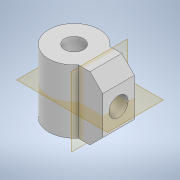
# Autodesk Inventor part: joint
Saved by Autodesk Inventor 2021 (Build 250183000, 183)
## iProperties
Created: 2020-12-08
Part Number: joint
Material: Generic
Document SubType Name: Modeling
Designer: awitc
Density: 1 g/cm^3
Appearance: Default
Author: awitc
Autodesk Inventor part; units mm, degrees
ref_plane "XY Plane" through (0, 0, 0) normal (0, 0, 1) x (1, 0, 0)
sketch "Sketch1" plane through (0, 0, 0) normal (0, 1, 0) x (-1, 0, 0)
  circle A0 centre (0, 0) radius 4
  circle A1 centre (0, 0) radius 1.5
  dimension "d0" = 8
  dimension "d1" = 3
  constraints: 2 centre point, 2 coincident
  measures "d0" diameter of A0
  measures "d1" diameter of A1
extrude "Extrusion1" add sketch "Sketch1" along normal blind 10
ref_plane "Work Plane1" through (4, 0, 0) normal (1, 0, 0) x (0, 1, 0)
sketch "Sketch2" plane through (4, 0, 0) normal (1, 0, 0) x (0, 1, 0)
  line L0 (0, -4) -> (10, -4) projected
  line L1 (10, -4) -> (10, 4) projected
  line L2 (0, -4) -> (10, -4)
  line L3 (10, -4) -> (10, 4)
  line L4 (10, 4) -> (0, 4)
  line L5 (0, 4) -> (0, -4)
  line L6 (0, 0) -> (0, 2.5)
  line L7 (0, -4) -> (0, 4) projected
  line L8 (0, 2.5) -> (0, -2.5)
  line L9 (0, -2.5) -> (10, -2.5)
  line L10 (0, 2.5) -> (10, 2.5)
  dimension "d5" = 2.5
  dimension "d6" = 5
  constraints: 16 end point, 5 point on line, 3 perpendicular, 2 parallel, 1 horizontal
  measures "d5" distance of L6.start L6.end
  measures "d6" distance of L6.end L8.end
extrude "Extrusion2" add sketch "Sketch2" along normal blind 3 and the other way blind 2.5 contours L5 L10 L1 L9
sketch "Sketch3" plane through (7, 0, 0) normal (1, 0, 0) x (0, 0, -1)
  line L0 (0, 0) -> (0, 10)
  line L1 (4, 10) -> (-4, 10) projected
  circle A0 centre (0, 5) radius 1.5
  point P0 (2.5, 10)
  point P1 (-2.5, 10)
  dimension "d11" = 3
  constraints: 2 end point, 2 midpoint, 1 centre point
  measures "d11" diameter of A0
extrude "Extrusion3" cut sketch "Sketch3" against normal blind 5
ref_plane "Work Plane2" through (0, 5, 0) normal (0, 1, 0) x (-1, 0, 0)
chamfer "Chamfer2" distance 2 angle 45 2 edges at (7, 10, 0) (7, 0, 0)
body "Solid1"
